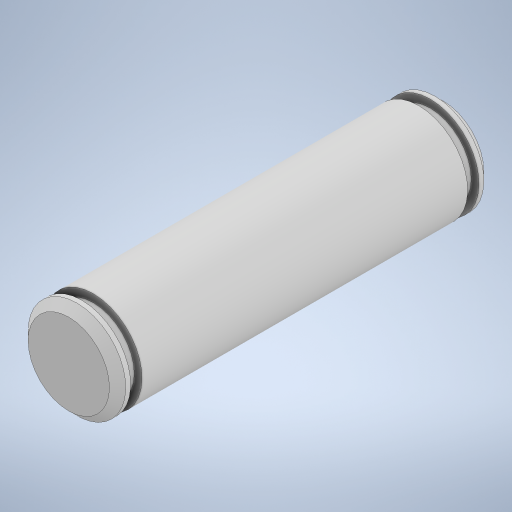
# Autodesk Inventor part: D6 L20 rod pin
Saved by Autodesk Inventor 2023 (Build 270158000, 158)
## iProperties
Created: 2023-02-24
Part Number: D6 L20 rod pin
Material: Generic
Document SubType Name: Modeling
Designer: roota
Density: 1 g/cm^3
Appearance: Default
Author: roota
Autodesk Inventor part; units mm, degrees
ref_plane "YZ Plane" through (0, 0, 0) normal (1, 0, 0) x (0, 1, 0)
ref_plane "XZ Plane" through (0, 0, 0) normal (0, 1, 0) x (-1, 0, 0)
ref_plane "XY Plane" through (0, 0, 0) normal (0, 0, 1) x (1, 0, 0)
sketch "Sketch1" plane through (0, 0, 0) normal (1, 0, 0) x (0, 1, 0)
  line L0 (0, 0) -> (3, 0)
  line L1 (3, 0) -> (3, -23)
  line L2 (3, -23) -> (0, -23)
  line L3 (0, -23) -> (0, 0)
  line L4 (3, -0.8) -> (2.525, -0.8)
  line L5 (2.525, -0.8) -> (2.525, -1.5)
  line L6 (2.525, -1.5) -> (3, -1.5)
  line L7 (3, -1.5) -> (3, -0.8)
  line L8 (3, -22.2) -> (2.525, -22.2)
  line L9 (2.525, -22.2) -> (2.525, -21.5)
  line L10 (2.525, -21.5) -> (3, -21.5)
  line L11 (3, -21.5) -> (3, -22.2)
  point P0 (2.525, -21.85)
  point P1 (3, -21.5)
  point P2 (1.5, -23)
  dimension "d0" = 6
  dimension "d1" = 20
  dimension "d4" = 0.7
  dimension "d5" = 0.7
  dimension "d6" = 5.05
  dimension "d11" = 23
  dimension "d12" = 0.8
  constraints: 24 end point, 6 parallel, 3 horizontal, 3 perpendicular, 3 point on line, 2 midpoint, 1 vertical alignment
  measures "d0" diameter of L1 L3
  measures "d1" distance between parallel lines of L10 L6
  measures "d4" distance of L4.end L5.end
  measures "d5" distance of L8.end L9.end
  measures "d6" diameter of point (2.525, -21.85) L3
  measures "d11" distance from line of point (1.5, -23) L0
  measures "d12" distance of L0.end L4.start
revolve "Revolution1" add sketch "Sketch1" angle 360 about axis through (0, 0, -23) along (0, 0, 1) contours L0 L1 L4 L5 L6 L10 L9 L8 L2 L3
chamfer "Chamfer1" distance 0.5 angle 45 2 edges at (0, -3, 0) (0, -3, -23)
equation "\"d5\" = d4"
body "Solid1"
